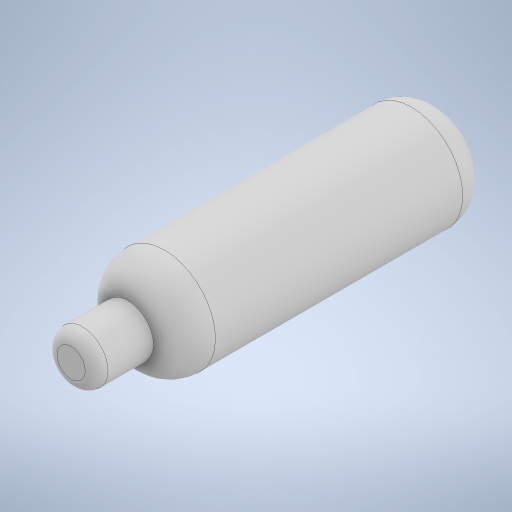
# Autodesk Inventor part: 8g_CO2_Cylinder
Saved by Autodesk Inventor 2023 (Build 270158000, 158)
## iProperties
Created: 2023-01-26
Part Number: 8g_CO2_Cylinder
Material: Generic
Document SubType Name: Modeling
Designer: Kuba
Density: 1 g/cm^3
Appearance: Default
Author: Kuba
Autodesk Inventor part; units mm, degrees
ref_plane "YZ Plane" through (0, 0, 0) normal (1, 0, 0) x (0, 1, 0)
ref_plane "XZ Plane" through (0, 0, 0) normal (0, 1, 0) x (-1, 0, 0)
ref_plane "XY Plane" through (0, 0, 0) normal (0, 0, 1) x (1, 0, 0)
sketch "Sketch1" plane through (0, 0, 0) normal (0, 0, 1) x (1, 0, 0)
  circle A0 centre (0, 0) radius 9
  circle A1 centre (0, 0) radius 4.5
  dimension "d0" = 18
  dimension "d1" = 9
  constraints: 2 centre point, 2 coincident
  measures "d0" diameter of A0
  measures "d1" diameter of A1
extrude "Extrusion1" add sketch "Sketch1" along normal blind 55 contours A0 | A1
sketch "Sketch2" plane through (0, 0, 55) normal (0, 0, 1) x (1, 0, 0)
  circle A0 centre (0, 0) radius 4.5
  dimension "d4" = 9
  constraints: 1 centre point, 1 coincident
  measures "d4" diameter of A0
extrude "Extrusion2" add sketch "Sketch2" along normal blind 10
fillet "Fillet1" radius 6.7625 1 edges at (-9, 0, 55)
fillet "Fillet2" radius 2 1 edges at (-4.5, 0, 65)
fillet "Fillet3" radius 5.175 1 edges at (-9, 0, 0)
body "Solid1"
